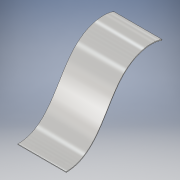
# Autodesk Inventor part: Bent_Plate
Saved by Autodesk Inventor 2019 (Build 230136000, 136)
## iProperties
Created: 2019-01-06
Part Number: Bent_Plate
Material: Generic
Document SubType Name: Modeling
Designer: Taran Mayer
Density: 1 g/cm^3
Appearance: Aluminum - Dark
Author: Taran Mayer
Autodesk Inventor part; units mm, degrees
ref_plane "YZ Plane" through (0, 0, 0) normal (1, 0, 0) x (0, 1, 0)
ref_plane "XZ Plane" through (0, 0, 0) normal (0, 1, 0) x (-1, 0, 0)
ref_plane "XY Plane" through (0, 0, 0) normal (0, 0, 1) x (1, 0, 0)
sketch "Sketch1" plane through (0, 0, 0) normal (1, 0, 0) x (0, 1, 0)
  line L0 (0, 0) -> (0, -27.2586) construction
  line L1 (0, -27.2586) -> (38.6099, -56.4871) construction
  line L2 (38.6099, -56.4871) -> (92.4517, -69.1015) construction
  line L3 (92.4517, -69.1015) -> (92.4517, -116.1747) construction
  line L4 (92.4517, -116.1747) -> (87.6906, -126.6322) construction
  spline S0 degree 4 poles (0, 0) (0, -27.2586) (38.6099, -56.4871) (92.4517, -69.1015) (92.4517, -116.1747) (87.6906, -126.6322) knots 1 1 1 1 1 2 3 3 3 3 3
  line L5 (-0.9769, -0.1832) -> (-0.9769, -27.4418) construction
  line L6 (-0.9769, -27.4418) -> (37.6329, -56.6703) construction
  line L7 (37.6329, -56.6703) -> (91.4748, -69.2847) construction
  line L8 (91.4748, -69.2847) -> (91.4748, -116.3578) construction
  line L9 (91.4748, -116.3578) -> (86.6272, -126.148) construction
  spline S1 degree 4 poles (-0.9769, -0.1832) (-0.9769, -27.4418) (37.6329, -56.6703) (91.4748, -69.2847) (91.4748, -116.3578) (86.6272, -126.148) knots 1 1 1 1 1 2 3 3 3 3 3
  line L10 (87.6906, -126.6322) -> (86.6272, -126.148)
  line L11 (0, 0) -> (-0.9769, -0.1832)
  dimension "d2" = 1.1684
  constraints: 4 end point, 2 vertical, 1 perpendicular, 6 other
  measures "d2" distance of L4.end L9.end
extrude "Extrusion1" add sketch "Sketch1" along normal blind 63.5
equation "\"BendRadius\" = Thickness"
equation "\"BendReliefWidth\" = Thickness"
equation "\"BendReliefDepth\" = 0.5 * Thickness"
equation "\"CornerReliefSize\" = 4 * Thickness"
equation "\"MinimumRemnant\" = 2 * Thickness"
equation "\"TransitionRadius\" = BendRadius"
equation "\"JacobiRadiusSize\" = Thickness"
equation "\"GapSize\" = Thickness"
equation "\"Thickness\" = 3.048"
body "Solid1"
